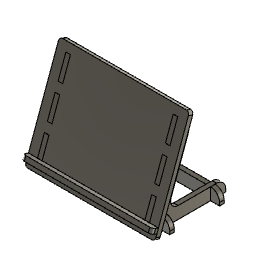
Flat-Pack-Easel (Autodesk Fusion 360 design; units mm, degrees)
Autodesk Fusion 360 part; units mm, degrees
sketch "Sketch1" plane through (0, 0, 0) normal (0, 1, 0) x (1, 0, 0)
  line L0 (-215, -155) -> (215, -155)
  line L1 (215, -155) -> (215, 155)
  line L2 (215, 155) -> (-215, 155)
  line L3 (-215, 155) -> (-215, -155)
  line L4 (-215, -155) -> (215, 155) construction
  line L5 (215, -155) -> (-215, 155) construction
  dimension "d1" = 310
  dimension "d2" = 430
  constraint horizontal L0
  constraint perpendicular L0 L1
  constraint parallel L0 L2
  constraint parallel L1 L3
  constraint coincident L4 origin
  constraint coincident L5 origin
  measures "d1" distance of L0.end L1.end
  measures "d2" distance of L0.start L0.end
extrude "Extrude1" add sketch "Sketch1" against normal blind 15 makes body 1
extrude "Extrude2" add 1 faces at (71.6667, -5, -155) along direction (0, 0, -1) blind 25 on bodies 1 bodies 1
sketch "Sketch2" plane through (0, -15, 0) normal (0, -1, 0) x (1, 0, 0)
  line L0 (-215, 155) -> (-215, -180)
  line L1 (-215, -180) -> (215, -180)
  line L2 (215, -180) -> (215, 155)
  line L3 (215, 155) -> (-215, 155)
  line L4 (-215, -145) -> (215, -145)
  line L5 (215, -145) -> (215, -160)
  line L6 (215, -160) -> (-215, -160)
  line L7 (-215, -160) -> (-215, -145)
  dimension "d8" = 15
  dimension "d9" = 20
  constraint horizontal L4
  constraint vertical L5
  constraint horizontal L6
  constraint vertical L7
  constraint coincident L2 L5.end
  constraint coincident L0 L4.start
  measures "d8" distance of L4.start L6.end
  measures "d9" distance of L1 L6
copy_body "Body->Comp1" bodies 1 removing the originals makes body 2 in component "Component"
extrude "Extrude1'" add sketch "Sketch2" along normal blind 20 separate body contours L0 L2 L4 L5 L6 L7 makes body 3 in component "Component'"
sketch "Sketch4" plane through (0, -15, 0) normal (0, 1, 0) x (-1, 0, 0)
  line L0 (-215, -160) -> (215, -160)
  line L1 (215, -160) -> (215, -145)
  line L2 (215, -145) -> (-215, -145)
  line L3 (-215, -145) -> (-215, -160)
  line L4 (-170, -145) -> (-95, -145)
  line L5 (-95, -145) -> (-95, -160)
  line L6 (-95, -160) -> (-170, -160)
  line L7 (-170, -160) -> (-170, -145)
  line L8 (170, -145) -> (95, -145)
  line L9 (170, -160) -> (170, -145)
  line L10 (95, -160) -> (170, -160)
  line L11 (95, -145) -> (95, -160)
  line L12 (215, -180) -> (215, 155)
  line L13 (-37.5, -145) -> (37.5, -145)
  line L14 (37.5, -145) -> (37.5, -160)
  line L15 (37.5, -160) -> (-37.5, -160)
  line L16 (-37.5, -160) -> (-37.5, -145)
  line L17 (0, -145) -> (0, -160) construction
  dimension "d12" = 75
  dimension "d13" = 45
  dimension "d53" = 45
  dimension "d54" = 75
  dimension "d55" = 15
  dimension "d56" = 15
  dimension "d57" = 75
  dimension "d58" = 215
  constraint horizontal L4
  constraint vertical L5
  constraint horizontal L6
  constraint vertical L7
  constraint coincident L0 L5.end
  constraint coincident L2 L4.start
  constraint parallel L8 L10
  constraint parallel L9 L11
  constraint perpendicular L10 L11
  constraint collinear L6 L10
  constraint horizontal L13
  constraint vertical L14
  constraint horizontal L15
  constraint vertical L16
  constraint coincident L0 L14.end
  constraint midpoint L13 L17.start
  constraint midpoint L15 L17.end
  measures "d12" distance of L4.start L4.end
  measures "d13" distance of L3 L7
  measures "d53" distance of L9 L12
  measures "d54" distance of L8.start L8.end
  measures "d55" distance of L8.start L9.start
  measures "d56" distance of L13.start L15.end
  measures "d57" distance of L13.start L13.end
  measures "d58" distance of L3 L17
extrude "Extrude2'" add sketch "Sketch4" along normal blind 15 contours L0 L2 L4 L5 L6 L7 | L0 L2 L13 L14 L15 L16 | L0 L2 L8 L9 L10 L11 bodies 3 in component "Component'"
combine "Combine1" operation cut target body 2 tool bodies 3 keep tools in component "Component"
sketch "Sketch5" plane through (0, 0, 0) normal (0, 1, 0) x (-1, 0, 0)
  line L0 (37.5, -160) -> (-37.5, -160)
  line L1 (-37.5, -145) -> (37.5, -145)
  line L2 (215, -180) -> (215, 155)
  line L3 (215, 155) -> (-215, 155)
  line L4 (-215, 155) -> (-215, -180)
  line L5 (-215, -180) -> (215, -180)
  line L6 (-185, 155) -> (-170, 155)
  line L7 (-170, 155) -> (-170, -180)
  line L8 (-170, -180) -> (-185, -180)
  line L9 (-185, -180) -> (-185, 155)
  line L10 (95, -160) -> (95, -145)
  line L11 (170, -145) -> (170, -160)
  line L12 (-95, -145) -> (-95, -160)
  line L13 (-95, -160) -> (-170, -160)
  line L14 (-170, -160) -> (-170, -145)
  line L15 (-170, -145) -> (-95, -145)
  line L16 (37.5, -145) -> (37.5, -160)
  line L17 (-37.5, -160) -> (-37.5, -145)
  line L18 (95, -145) -> (170, -145)
  line L19 (170, -160) -> (95, -160)
  dimension "d16" = 15
  dimension "d17" = 30
  constraint horizontal L6
  constraint vertical L7
  constraint horizontal L8
  constraint vertical L9
  constraint coincident L5 L7.end
  constraint coincident L3 L6.start
  measures "d16" distance of L6.start L6.end
  measures "d17" distance of L4 L9
extrude "Extrude1''" add sketch "Sketch5" along normal blind 40 separate body contours L3 L5 L6 L7 L8 L9 L14 makes body 4 in component "Component''"
move_body "Move1" bodies 4 to x (1, 0, 0) y (0, 0.939693, -0.34202) z (0, 0.34202, 0.939693) at (0, 61.5636, -10.8553) in component "Component''"
move_body "Move1'" bodies 3 to x (1, 0, 0) y (0, 0.939693, -0.34202) z (0, 0.34202, 0.939693) at (0, 61.5636, -10.8553) in component "Component'"
move_body "Move1''" bodies 2 to x (1, 0, 0) y (0, 0.939693, -0.34202) z (0, 0.34202, 0.939693) at (0, 61.5636, -10.8553) in component "Component"
sketch "Sketch6" plane through (185, 0, 0) normal (1, 0, 0) x (0, 1, 0)
  line L0 (114.5767, 134.797) -> (0, -180)
  line L1 (0, -180) -> (37.5877, -193.6808)
  line L2 (37.5877, -193.6808) -> (152.1645, 121.1162)
  line L3 (152.1645, 121.1162) -> (114.5767, 134.797)
  line L4 (0, -180) -> (250, -180)
  line L5 (250, -180) -> (250, -140)
  line L6 (250, -140) -> (57.1259, -140)
  arc A0 (124.6305, 45.4674) -> (114.5767, 134.797) centre (29.7115, 80.0151) ccw
  dimension "d23" = 40
  dimension "d24" = 250
  constraint horizontal L4
  constraint vertical L5
  constraint horizontal L6
  constraint coincident L0.end L1.start
  constraint coincident L2 L6.end
  constraint tangent L2 A0
  constraint coincident L2 A0.start
  constraint coincident L0.start L3.end
  measures "d23" distance of L4.end L5.end
  measures "d24" distance of L0.end L4.end
extrude "Extrude2''" add sketch "Sketch6" against normal blind 15 contours L2 L4 L5 L6 bodies 4 in component "Component''"
extrude "Extrude3" cut sketch "Sketch6" against normal blind 25 contours L2 L3 A0 | L1 L2 L4 bodies 4 in component "Component''"
sketch "Sketch7" plane through (0, 57.8509, -21.056) normal (0, -0.939693, 0.34202) x (1, 0, 0)
  line L0 (185, -169.1447) -> (185, 165.8553)
  line L1 (170, 165.8553) -> (170, -169.1447)
  line L2 (170, 139.6053) -> (185, 139.6053)
  line L3 (185, 139.6053) -> (185, 64.6053)
  line L4 (185, 64.6053) -> (170, 64.6053)
  line L5 (170, 64.6053) -> (170, 139.6053)
  line L6 (170, 35.8553) -> (185, 35.8553)
  line L7 (185, 35.8553) -> (185, -39.1447)
  line L8 (185, -39.1447) -> (170, -39.1447)
  line L9 (170, -39.1447) -> (170, 35.8553)
  line L10 (170, -1.6447) -> (185, -1.6447) construction
  line L11 (170, -142.8947) -> (185, -142.8947)
  line L12 (170, -67.8947) -> (170, -142.8947)
  line L13 (185, -67.8947) -> (170, -67.8947)
  line L14 (185, -142.8947) -> (185, -67.8947)
  line L15 (185, 165.8553) -> (170, 165.8553)
  line L16 (170, 102.1053) -> (185, 102.1053) construction
  dimension "d29" = 75
  dimension "d59" = 75
  dimension "d78" = 66.25
  constraint horizontal L2
  constraint vertical L3
  constraint horizontal L4
  constraint vertical L5
  constraint coincident L0 L3.end
  constraint coincident L1 L2.start
  constraint horizontal L6
  constraint vertical L7
  constraint horizontal L8
  constraint vertical L9
  constraint coincident L0 L7.end
  constraint coincident L1 L6.start
  constraint midpoint L0 L7
  constraint midpoint L9 L10.start
  constraint midpoint L7 L10.end
  constraint symmetric L2.start L10 L11.start
  constraint symmetric L2.end L10 L11.end
  constraint symmetric L3.end L10 L13.start
  constraint symmetric L4.end L10 L12.start
  constraint midpoint L5 L16.start
  constraint midpoint L3 L16.end
  measures "d29" distance of L2.end L3.end
  measures "d59" distance of L6.end L7.end
  measures "d78" distance of L6 L16
extrude "Extrude4" add sketch "Sketch7" along normal blind 15 contours L0 L1 L11 L12 L13 L14 | L0 L1 L6 L7 L8 L9 | L0 L1 L2 L3 L4 L5 bodies 4 in component "Component''"
mirror "Mirror1" about plane through (0, 0, 0) normal (1, 0, 0) of bodies 4 makes body 5 in component "Component''"
combine "Combine2" operation cut target body 2 tool bodies 5 4 keep tools in component "Component"
fillet "Fillet1" radius 10 4 edges at (-215, 107.5291, 137.3622) (215, 107.5291, 137.3622) (215, -7.0477, -177.4348) (-215, -7.0477, -177.4348) on bodies 2 in component "Component"
fillet "Fillet1'" radius 10 2 edges at (-215, -23.4837, -142.1877) (215, -23.4837, -142.1877) on bodies 3 in component "Component'"
fillet "Fillet1''" radius 25 2 edges at (177.5, 57.1259, -140) (-177.5, 57.1259, -140) on bodies 4 5 in component "Component''"
sketch "Sketch8" plane through (0, 43.7555, -15.9257) normal (0, -0.939693, 0.34202) x (1, 0, 0)
  line L0 (-170, -134.1447) -> (-95, -134.1447)
  line L1 (215, -159.1447) -> (215, 155.8553)
  arc A0 (215, 155.8553) -> (205, 165.8553) centre (205, 155.8553) ccw
  line L2 (205, 165.8553) -> (-205, 165.8553)
  arc A1 (-205, 165.8553) -> (-215, 155.8553) centre (-205, 155.8553) ccw
  line L3 (-215, 155.8553) -> (-215, -159.1447)
  line L4 (-95, -134.1447) -> (-95, -149.1447)
  line L5 (-95, -149.1447) -> (-170, -149.1447)
  line L6 (170, -142.8947) -> (170, -149.1447)
  line L7 (170, -149.1447) -> (95, -149.1447)
  line L8 (95, -149.1447) -> (95, -134.1447)
  line L9 (-170, 64.6053) -> (-185, 64.6053)
  line L10 (-185, 64.6053) -> (-185, 139.6053)
  line L11 (-185, 139.6053) -> (-170, 139.6053)
  line L12 (-170, 139.6053) -> (-170, 64.6053)
  line L13 (185, 64.6053) -> (170, 64.6053)
  line L14 (170, 64.6053) -> (170, 139.6053)
  line L15 (170, 139.6053) -> (185, 139.6053)
  line L16 (185, 139.6053) -> (185, 64.6053)
  arc A2 (-215, -159.1447) -> (-205, -169.1447) centre (-205, -159.1447) ccw
  line L17 (-205, -169.1447) -> (205, -169.1447)
  arc A3 (205, -169.1447) -> (215, -159.1447) centre (205, -159.1447) ccw
  line L18 (37.5, -134.1447) -> (37.5, -149.1447)
  line L19 (37.5, -149.1447) -> (-37.5, -149.1447)
  line L20 (-37.5, -149.1447) -> (-37.5, -134.1447)
  line L21 (-37.5, -134.1447) -> (37.5, -134.1447)
  line L22 (-170, -149.1447) -> (-170, -142.8947)
  line L23 (-185, -67.8947) -> (-170, -67.8947)
  line L24 (-170, -67.8947) -> (-170, -134.1447)
  line L25 (-170, -142.8947) -> (-185, -142.8947)
  line L26 (-185, -142.8947) -> (-185, -67.8947)
  line L27 (-170, -39.1447) -> (-185, -39.1447)
  line L28 (-185, -39.1447) -> (-185, 35.8553)
  line L29 (-185, 35.8553) -> (-170, 35.8553)
  line L30 (-170, 35.8553) -> (-170, -39.1447)
  line L31 (170, -67.8947) -> (185, -67.8947)
  line L32 (185, -67.8947) -> (185, -142.8947)
  line L33 (185, -142.8947) -> (170, -142.8947)
  line L34 (185, -39.1447) -> (170, -39.1447)
  line L35 (170, -39.1447) -> (170, 35.8553)
  line L36 (170, 35.8553) -> (185, 35.8553)
  line L37 (185, 35.8553) -> (185, -39.1447)
  line L38 (95, -134.1447) -> (170, -134.1447)
  line L39 (170, -134.1447) -> (170, -67.8947)
sketch "Sketch9" plane through (-185, 0, 0) normal (-1, 0, 0) x (0, -1, 0)
  line L0 (-79.9472, 39.6532) -> (-65.8518, 44.7835)
  line L1 (5.1174, -150.2028) -> (-20.5342, -79.7258)
  line L2 (-91.5033, 115.2604) -> (-105.5987, 110.1301)
  line L3 (-250, -180) -> (0, -180)
  line L4 (0, -180) -> (-8.978, -155.3331)
  line L5 (-8.978, -155.3331) -> (5.1174, -150.2028)
  line L6 (-20.5342, -79.7258) -> (-34.6295, -84.8561)
  line L7 (-34.6295, -84.8561) -> (-44.4626, -57.84)
  line L8 (-44.4626, -57.84) -> (-30.3672, -52.7097)
  line L9 (-30.3672, -52.7097) -> (-56.0187, 17.7673)
  line L10 (-56.0187, 17.7673) -> (-70.1141, 12.637)
  line L11 (-70.1141, 12.637) -> (-79.9472, 39.6532)
  line L12 (-105.5987, 110.1301) -> (-114.5767, 134.797)
  arc A0 (-114.5767, 134.797) -> (-124.6305, 45.4674) centre (-29.7115, 80.0151) ccw
  line L13 (-124.6305, 45.4674) -> (-69.3373, -106.4495)
  arc A1 (-92.8296, -140) -> (-69.3373, -106.4495) centre (-92.8296, -115) ccw
  line L14 (-92.8296, -140) -> (-250, -140)
  line L15 (-250, -140) -> (-250, -180)
  line L16 (-65.8518, 44.7835) -> (-91.5033, 115.2604)
sketch "Sketch10" plane through (0, -45.8802, -126.0548) normal (0, 0.34202, 0.939693) x (-1, 0, 0)
  arc A0 (-205, -26.5636) -> (-215, -36.5636) centre (-205, -36.5636) ccw
  line L0 (-215, -36.5636) -> (-215, -46.5636)
  line L1 (-170, -61.5636) -> (-95, -61.5636)
  line L2 (215, -46.5636) -> (215, -36.5636)
  arc A1 (215, -36.5636) -> (205, -26.5636) centre (205, -36.5636) ccw
  line L3 (205, -26.5636) -> (-205, -26.5636)
  line L4 (-215, -46.5636) -> (-170, -46.5636)
  line L5 (-170, -46.5636) -> (-170, -61.5636)
  line L6 (-95, -61.5636) -> (-95, -46.5636)
  line L7 (37.5, -46.5636) -> (95, -46.5636)
  line L8 (95, -46.5636) -> (95, -61.5636)
  line L9 (95, -61.5636) -> (170, -61.5636)
  line L10 (170, -61.5636) -> (170, -46.5636)
  line L11 (170, -46.5636) -> (215, -46.5636)
  line L12 (-95, -46.5636) -> (-37.5, -46.5636)
  line L13 (-37.5, -46.5636) -> (-37.5, -61.5636)
  line L14 (-37.5, -61.5636) -> (37.5, -61.5636)
  line L15 (37.5, -61.5636) -> (37.5, -46.5636)
sketch "Sketch11" plane through (0, 0, -180) normal (0, 0, -1) x (1, 0, 0)
  line L0 (185, -250) -> (185, 0)
  line L1 (170, 0) -> (170, -250)
  line L2 (215, -35) -> (-215, -35)
  line L3 (-215, -35) -> (-215, -50)
  line L4 (-215, -50) -> (215, -50)
  line L5 (215, -50) -> (215, -35)
  line L6 (-205, 0) -> (205, 0)
  line L7 (0, 0) -> (0, -35)
  line L8 (185, -125) -> (170, -125) construction
  line L9 (215, -215) -> (-215, -215)
  line L10 (-215, -200) -> (215, -200)
  line L11 (215, -200) -> (215, -215)
  line L12 (-215, -215) -> (-215, -200)
  line L13 (170, -250) -> (185, -250)
  line L14 (185, 0) -> (170, 0)
  dimension "d60" = 430
  dimension "d61" = 15
  dimension "d62" = 35
  constraint horizontal L2
  constraint vertical L3
  constraint horizontal L4
  constraint vertical L5
  constraint coincident L7.start origin
  constraint midpoint L2 L7.end
  constraint vertical L7
  constraint midpoint L0 L8.start
  constraint midpoint L1 L8.end
  constraint symmetric L2.start L8 L9.start
  constraint symmetric L2.end L8 L9.end
  constraint symmetric L3.end L8 L10.start
  constraint symmetric L4.end L8 L10.end
  measures "d60" distance of L3.end L4.end
  measures "d61" distance of L2.start L4.end
  measures "d62" distance of L2 L6
extrude "Extrude1'''" add sketch "Sketch11" against normal blind 40 separate body contours L0 L1 L2 L4 | L0 L2 L4 L5 | L1 L2 L3 L4 makes body 6 in component "Component'''"
extrude "Extrude1''''" add sketch "Sketch11" against normal blind 40 separate body contours L0 L1 L9 L10 | L0 L9 L10 L11 | L1 L9 L10 L12 makes body 7 in component "Component''''"
sketch "Sketch12" plane through (0, 50, 0) normal (0, 1, 0) x (-1, 0, 0)
  line L0 (215, -180) -> (215, -140)
  line L1 (215, -140) -> (-215, -140)
  line L2 (-215, -140) -> (-215, -180)
  line L3 (-185, -160) -> (-215, -160) construction
  line L4 (-185, -160) -> (-170, -160)
  line L5 (-170, -160) -> (-170, -140)
  line L6 (-170, -140) -> (-185, -140)
  line L7 (-185, -140) -> (-185, -160)
  line L8 (0, 20) -> (0, 2.5)
  line L9 (185, -140) -> (185, -160)
  line L10 (170, -140) -> (185, -140)
  line L11 (170, -160) -> (170, -140)
  line L12 (185, -160) -> (170, -160)
  line L13 (-185, 39.6532) -> (-185, 44.7835)
  line L14 (-170, 39.6532) -> (-170, 44.7835)
  line L15 (-170, 115.2604) -> (-170, 44.7835)
  line L16 (-185, -57.84) -> (-185, -52.7097)
  line L17 (-170, -57.84) -> (-170, -52.7097)
  line L18 (-170, -57.84) -> (-170, -79.7258)
  line L19 (-185, -79.7258) -> (-185, -57.84)
  line L20 (-185, -155.3331) -> (-185, -150.2028)
  line L21 (-170, -155.3331) -> (-170, -150.2028)
  line L22 (-185, -150.2028) -> (-185, -79.7258)
  line L23 (-170, -79.7258) -> (-170, -150.2028)
  line L24 (-170, -155.3331) -> (-170, -180)
  line L25 (-170, -180) -> (-185, -180)
  line L26 (-185, -180) -> (-185, -155.3331)
  line L27 (-185, 17.7673) -> (-185, 39.6532)
  line L28 (-170, 39.6532) -> (-170, 17.7673)
  line L29 (-185, 44.7835) -> (-185, 115.2604)
  line L30 (-185, 134.797) -> (-170, 134.797)
  line L31 (-185, 115.2604) -> (-185, 134.797)
  line L32 (-170, 134.797) -> (-170, 115.2604)
  line L33 (-185, -52.7097) -> (-185, 17.7673)
  line L34 (-170, 17.7673) -> (-170, -52.7097)
  dimension "d81" = 30
  dimension "d82" = 15
  constraint midpoint L2 L3.end
  constraint horizontal L3
  constraint horizontal L4
  constraint vertical L5
  constraint horizontal L6
  constraint vertical L7
  constraint coincident L1 L5.end
  constraint symmetric L3.start L8 L9.end
  constraint symmetric L4.end L8 L11.start
  constraint symmetric L5.end L8 L10.start
  constraint symmetric L6.end L8 L9.start
  measures "d81" distance of L2 L7
  measures "d82" distance of L5 L7
extrude "Extrude2'''" cut sketch "Sketch12" against normal blind 25 contours L1 L9 L10 L11 L12 | L1 L4 L5 L6 L7 L20 L21 L22 L23 L24 L26 bodies 6 in component "Component'''"
combine "Combine1'" operation cut target body 5 tool bodies 6 keep tools in component "Component''"
combine "Combine2'" operation cut target body 4 tool bodies 6 keep tools in component "Component''"
sketch "Sketch13" plane through (0, 215, 0) normal (0, 1, 0) x (-1, 0, 0)
  line L0 (-215, -180) -> (215, -180)
  line L1 (215, -180) -> (215, -140)
  line L2 (215, -140) -> (-215, -140)
  line L3 (-215, -140) -> (-215, -180)
  line L4 (-170, 39.6532) -> (-170, 44.7835)
  line L5 (-170, 115.2604) -> (-170, 44.7835)
  line L6 (-185, 39.6532) -> (-185, 44.7835)
  line L7 (-185, -140) -> (-170, -140)
  line L8 (-170, -140) -> (-170, -160)
  line L9 (-170, -160) -> (-185, -160)
  line L10 (-185, -160) -> (-185, -140)
  line L11 (-185, -160) -> (-215, -160) construction
  line L12 (0, 20) -> (0, 2.5)
  line L13 (185, -160) -> (185, -140)
  line L14 (185, -140) -> (170, -140)
  line L15 (170, -140) -> (170, -160)
  line L16 (170, -160) -> (185, -160)
  line L17 (-185, 115.2604) -> (-185, 134.797)
  line L18 (-185, 17.7673) -> (-185, 39.6532)
  line L19 (-185, -52.7097) -> (-185, 17.7673)
  line L20 (-185, -57.84) -> (-185, -52.7097)
  line L21 (-185, -79.7258) -> (-185, -57.84)
  line L22 (-185, -150.2028) -> (-185, -79.7258)
  line L23 (-185, -155.3331) -> (-185, -150.2028)
  line L24 (-185, -180) -> (-185, -155.3331)
  line L25 (-170, -155.3331) -> (-170, -180)
  line L26 (-170, -155.3331) -> (-170, -150.2028)
  line L27 (-170, -57.84) -> (-170, -79.7258)
  line L28 (-170, -57.84) -> (-170, -52.7097)
  line L29 (-170, 17.7673) -> (-170, -52.7097)
  line L30 (-170, 39.6532) -> (-170, 17.7673)
  line L31 (-170, 134.797) -> (-170, 115.2604)
  line L32 (-170, -180) -> (-185, -180)
  line L33 (-185, 134.797) -> (-170, 134.797)
  line L34 (-185, 44.7835) -> (-185, 115.2604)
  line L35 (-170, -79.7258) -> (-170, -150.2028)
  dimension "d79" = 30
  dimension "d80" = 15
  constraint horizontal L7
  constraint vertical L8
  constraint horizontal L9
  constraint vertical L10
  constraint coincident L2 L7.start
  constraint midpoint L3 L11.end
  constraint horizontal L11
  constraint symmetric L7.start L12 L13.end
  constraint symmetric L7.end L12 L14.end
  constraint symmetric L8.end L12 L15.end
  constraint symmetric L9.end L12 L13.start
  measures "d79" distance of L3 L10
  measures "d80" distance of L8 L10
extrude "Extrude2''''" cut sketch "Sketch13" against normal blind 25 contours L2 L7 L8 L9 L10 L22 L23 L24 L25 L26 L35 | L2 L13 L14 L15 L16 bodies 7 in component "Component''''"
combine "Combine3" operation cut target body 4 tool bodies 7 keep tools in component "Component''"
combine "Combine4" operation cut target body 5 tool bodies 7 keep tools in component "Component''"
fillet "Fillet1'''" radius 30 2 edges at (215, 207.5, -140) (-215, 207.5, -140) on bodies 7 in component "Component''''"
fillet "Fillet1''''" radius 30 2 edges at (215, 42.5, -140) (-215, 42.5, -140) on bodies 6 in component "Component'''"
fillet "Fillet2" radius 30 2 edges at (177.5, 250, -140) (-177.5, 250, -140) on bodies 4 5 in component "Component''"
sketch "Sketch14" plane through (0, 43.7555, -15.9257) normal (0, -0.939693, 0.34202) x (1, 0, 0)
  line L0 (-95, -134.1447) -> (-95, -149.1447)
  line L1 (-95, -149.1447) -> (-170, -149.1447)
  line L2 (-170, -149.1447) -> (-170, -142.8947)
  line L3 (-170, -134.1447) -> (-95, -134.1447)
  line L4 (37.5, -134.1447) -> (37.5, -149.1447)
  line L5 (37.5, -149.1447) -> (-37.5, -149.1447)
  line L6 (-37.5, -149.1447) -> (-37.5, -134.1447)
  line L7 (-37.5, -134.1447) -> (37.5, -134.1447)
  line L8 (170, -142.8947) -> (170, -149.1447)
  line L9 (170, -149.1447) -> (95, -149.1447)
  line L10 (95, -149.1447) -> (95, -134.1447)
  line L11 (95, -134.1447) -> (170, -134.1447)
  line L12 (-170, 64.6053) -> (-185, 64.6053)
  line L13 (-185, 64.6053) -> (-185, 139.6053)
  line L14 (-185, 139.6053) -> (-170, 139.6053)
  line L15 (-170, 139.6053) -> (-170, 64.6053)
  line L16 (-185, -67.8947) -> (-170, -67.8947)
  line L17 (-170, -67.8947) -> (-170, -134.1447)
  line L18 (-170, -142.8947) -> (-185, -142.8947)
  line L19 (-185, -142.8947) -> (-185, -67.8947)
  line L20 (-170, -39.1447) -> (-185, -39.1447)
  line L21 (-185, -39.1447) -> (-185, 35.8553)
  line L22 (-185, 35.8553) -> (-170, 35.8553)
  line L23 (-170, 35.8553) -> (-170, -39.1447)
  line L24 (185, 64.6053) -> (170, 64.6053)
  line L25 (170, 64.6053) -> (170, 139.6053)
  line L26 (170, 139.6053) -> (185, 139.6053)
  line L27 (185, 139.6053) -> (185, 64.6053)
  line L28 (170, -67.8947) -> (185, -67.8947)
  line L29 (185, -67.8947) -> (185, -142.8947)
  line L30 (185, -142.8947) -> (170, -142.8947)
  line L31 (185, -39.1447) -> (170, -39.1447)
  line L32 (170, -39.1447) -> (170, 35.8553)
  line L33 (170, 35.8553) -> (185, 35.8553)
  line L34 (185, 35.8553) -> (185, -39.1447)
  arc A0 (-215, -159.1447) -> (-205, -169.1447) centre (-205, -159.1447) ccw
  line L35 (-205, -169.1447) -> (205, -169.1447)
  arc A1 (205, -169.1447) -> (215, -159.1447) centre (205, -159.1447) ccw
  line L36 (215, -159.1447) -> (215, 155.8553)
  arc A2 (215, 155.8553) -> (205, 165.8553) centre (205, 155.8553) ccw
  line L37 (205, 165.8553) -> (-205, 165.8553)
  arc A3 (-205, 165.8553) -> (-215, 155.8553) centre (-205, 155.8553) ccw
  line L38 (-215, 155.8553) -> (-215, -159.1447)
  line L39 (170, -134.1447) -> (170, -67.8947)
sketch "Support" plane through (-185, 0, 0) normal (-1, 0, 0) x (0, -1, 0)
  arc A0 (-220, -140) -> (-250, -170) centre (-220, -170) ccw
  line L0 (-250, -170) -> (-250, -180)
  line L1 (-250, -180) -> (-215, -180)
  line L2 (-215, -180) -> (-215, -160)
  line L3 (-215, -160) -> (-200, -160)
  line L4 (-200, -160) -> (-200, -180)
  line L5 (-200, -180) -> (-50, -180)
  line L6 (-50, -180) -> (-50, -160)
  line L7 (-50, -160) -> (-35, -160)
  line L8 (-35, -160) -> (-35, -180)
  line L9 (-35, -180) -> (0, -180)
  line L10 (0, -180) -> (-8.978, -155.3331)
  line L11 (-8.978, -155.3331) -> (5.1174, -150.2028)
  line L12 (5.1174, -150.2028) -> (-20.5342, -79.7258)
  line L13 (-20.5342, -79.7258) -> (-34.6295, -84.8561)
  line L14 (-34.6295, -84.8561) -> (-44.4626, -57.84)
  line L15 (-44.4626, -57.84) -> (-30.3672, -52.7097)
  line L16 (-30.3672, -52.7097) -> (-56.0187, 17.7673)
  line L17 (-56.0187, 17.7673) -> (-70.1141, 12.637)
  line L18 (-70.1141, 12.637) -> (-79.9472, 39.6532)
  line L19 (-79.9472, 39.6532) -> (-65.8518, 44.7835)
  line L20 (-65.8518, 44.7835) -> (-91.5033, 115.2604)
  line L21 (-91.5033, 115.2604) -> (-105.5987, 110.1301)
  line L22 (-105.5987, 110.1301) -> (-114.5767, 134.797)
  arc A1 (-114.5767, 134.797) -> (-124.6305, 45.4674) centre (-29.7115, 80.0151) ccw
  line L23 (-124.6305, 45.4674) -> (-69.3373, -106.4495)
  arc A2 (-92.8296, -140) -> (-69.3373, -106.4495) centre (-92.8296, -115) ccw
  line L24 (-92.8296, -140) -> (-220, -140)
sketch "Ledge" plane through (0, -45.8802, -126.0548) normal (0, 0.34202, 0.939693) x (-1, 0, 0)
  arc A0 (-205, -26.5636) -> (-215, -36.5636) centre (-205, -36.5636) ccw
  line L0 (-215, -36.5636) -> (-215, -46.5636)
  line L1 (-215, -46.5636) -> (-170, -46.5636)
  line L2 (-170, -46.5636) -> (-170, -61.5636)
  line L3 (-170, -61.5636) -> (-95, -61.5636)
  line L4 (-95, -61.5636) -> (-95, -46.5636)
  line L5 (-95, -46.5636) -> (-37.5, -46.5636)
  line L6 (-37.5, -46.5636) -> (-37.5, -61.5636)
  line L7 (-37.5, -61.5636) -> (37.5, -61.5636)
  line L8 (37.5, -61.5636) -> (37.5, -46.5636)
  line L9 (37.5, -46.5636) -> (95, -46.5636)
  line L10 (95, -46.5636) -> (95, -61.5636)
  line L11 (95, -61.5636) -> (170, -61.5636)
  line L12 (170, -61.5636) -> (170, -46.5636)
  line L13 (170, -46.5636) -> (215, -46.5636)
  line L14 (215, -46.5636) -> (215, -36.5636)
  arc A1 (215, -36.5636) -> (205, -26.5636) centre (205, -36.5636) ccw
  line L15 (205, -26.5636) -> (-205, -26.5636)
sketch "Support2" plane through (0, 215, 0) normal (0, 1, 0) x (-1, 0, 0)
  arc A0 (215, -170) -> (185, -140) centre (185, -170) ccw
  line L0 (185, -140) -> (185, -160)
  line L1 (185, -160) -> (170, -160)
  line L2 (170, -160) -> (170, -140)
  line L3 (170, -140) -> (-170, -140)
  line L4 (-170, -140) -> (-170, -160)
  line L5 (-170, -160) -> (-185, -160)
  line L6 (-185, -160) -> (-185, -140)
  arc A1 (-185, -140) -> (-215, -170) centre (-185, -170) ccw
  line L7 (-215, -170) -> (-215, -180)
  line L8 (-215, -180) -> (215, -180)
  line L9 (215, -180) -> (215, -170)
component "Component'" placed x (1, 0, 0) y (0, 1, 0) z (0, 0, 1) at (0, 0, 0)
component "Component''" placed x (1, 0, 0) y (0, 1, 0) z (0, 0, 1) at (0, 0, 0)
component "Component'''" placed x (1, 0, 0) y (0, 1, 0) z (0, 0, 1) at (0, 0, 0)
component "Component''''" placed x (1, 0, 0) y (0, 1, 0) z (0, 0, 1) at (0, 0, 0)
component "Component" placed x (1, 0, 0) y (0, 1, 0) z (0, 0, 1) at (0, 0, 0)
equation "d1 = height"
equation "d2 = length"
equation "thickness = 15 mm"
equation "d4 = -thickness"
equation "d6 = thickness + 10 mm"
equation "d8 = thickness"
equation "d12 = 5 * thickness"
equation "d13 = 3 * thickness"
equation "d14 = thickness"
equation "d16 = thickness"
equation "d17 = 2 * thickness"
equation "d18 = support"
equation "d23 = support"
equation "d24 = supportLength"
equation "d25 = -thickness"
equation "d29 = 5 * thickness"
equation "d35 = thickness"
equation "length = 430 mm"
equation "height = 310 mm"
equation "support = 40 mm"
equation "supportLength = 250 mm"
equation "d53 = 3 * thickness"
equation "d54 = 5 * thickness"
equation "d55 = thickness"
equation "d56 = thickness"
equation "d57 = 5 * thickness"
equation "d58 = length / 2"
equation "d59 = d29"
equation "d60 = length"
equation "d61 = thickness"
equation "d78 = ( height / 2 - 3 / 2 * thickness ) / 2"
equation "d79 = 2 * thickness"
equation "d80 = thickness"
equation "d81 = 2 * thickness"
equation "d82 = thickness"
